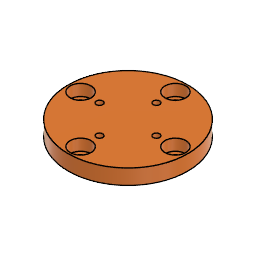
Assembly (Autodesk Fusion 360 archive; units mm, degrees)
design "Franka / UR10 mount"
part number: 2026-03-03-19-08-19-558
Autodesk Fusion 360 part; units mm, degrees
sketch "Sketch1" plane through (0, 0, 0) normal (0, 0, 1) x (1, 0, 0)
  circle A0 centre (0, 0) radius 15 construction
  circle A1 centre (0, 15) radius 1.7
  circle A2 centre (-15, 0) radius 1.7
  circle A3 centre (0, -15) radius 1.7
  circle A4 centre (15, 0) radius 1.7
  circle A5 centre (0, 0) radius 25
  circle A6 centre (0, 25) radius 1.5 construction
  circle A7 centre (-25, 0) radius 1.5 construction
  circle A8 centre (0, -25) radius 1.5 construction
  circle A9 centre (25, 0) radius 1.5 construction
  circle A10 centre (0, 0) radius 31.5
  circle A11 centre (0, 0) radius 25 construction
  dimension "d426" = 30
  dimension "d427" = 3.4
  dimension "d429" = 360
  dimension "d430" = 50
  dimension "d432" = 3
  dimension "d442" = 63
  dimension "d443" = 50
  constraint coincident A0.centre A5.centre
  constraint coincident A0 A1.centre
  constraint concentric A0 A5
  constraint coincident A5 A6.centre
  constraint concentric A5 A10
  constraint concentric A5 A11
  measures "d426" diameter of A0
  measures "d427" diameter of A1
  measures "d430" diameter of A5
  measures "d432" diameter of A6
  measures "d442" diameter of A10
  measures "d443" diameter of A11
extrude "Extrude1" add sketch "Sketch1" along normal blind 8 contours A5 | A10
hole "Hole2" at (15, 0, 0) at (0, -15, 0) at (-15, 0, 0) at (0, 15, 0) direction (0, 0, 1) diameter 3.4 depth 9 tip angle 118 counterbore diameter 6.5 counterbore depth 3
sketch "Sketch2" plane through (0, 0, 8) normal (0, 0, 1) x (-1, 0, 0)
  circle A0 centre (-15, 0) radius 1.7
  circle A1 centre (15, 0) radius 1.7
  circle A2 centre (0, 15) radius 1.7
  circle A3 centre (0, -15) radius 1.7
  circle A4 centre (0, 0) radius 31.5
  circle A5 centre (0, 0) radius 25
  circle A6 centre (0, -25) radius 1.5 construction
  circle A7 centre (25, 0) radius 1.5 construction
  circle A8 centre (0, 25) radius 1.5 construction
  circle A9 centre (-25, 0) radius 1.5 construction
  dimension "d449" = 50
  dimension "d450" = 3
  dimension "d452" = 360
  constraint coincident A4.centre A5.centre
  constraint coincident A5 A6.centre
  measures "d449" diameter of A5
  measures "d450" diameter of A6
hole "Hole3" at (0, 25, 8) at (25, 0, 8) at (0, -25, 8) at (-25, 0, 8) direction (0, 0, -1) diameter 6.6 depth 9 tip angle 118 counterbore diameter 11 counterbore depth 6
equation "d426 = promjer_utori"
equation "d443 = promjer_silikona"
equation "promjer_prihvata = promjer_silikona - 10 mm"
equation "promjer_silikona = 50 mm"
equation "promjer_utori = promjer_prihvata - 10 mm"
named bodies: "Franka prihvat"

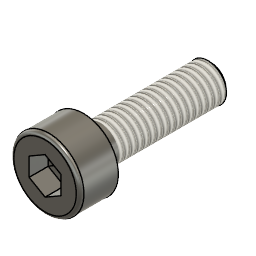
design "Broached Hexagon Socket Head Cap Screw ASME B18.3.1M - M3x0.5 x 10 Steel Grade 2 Plain"
description: Broached Hexagon Socket Head Cap Screw ASME B18.3.1M - M3x0.5 x 10
part number: BSHCS ASME B18.3.1M - M3x0.5 x 10 Steel Grade 2 Plain
Autodesk Fusion 360 part; units mm, degrees
sketch "Sketch1" plane through (0, 0, 0) normal (0, 1, 0) x (1, 0, 0)
  line L0 (-1.5, 0) -> (-1.5, 10)
  line L1 (-1.5, 10) -> (0, 10)
  line L2 (0, 10) -> (0, -3)
  line L3 (-1.5, 0) -> (-2.75, 0)
  line L4 (-2.75, 0) -> (-2.75, -3)
  line L5 (-2.75, -3) -> (0, -3)
  dimension "d101" = 10
  dimension "d102" = 3
  dimension "d109" = 5.5
  dimension "d110" = 3
  constraint perpendicular L0 L1
  constraint collinear origin L1.end L2.end
  constraint perpendicular L0 L3
  constraint coincident origin L3
  constraint vertical L2
  constraint coincident L2 L5.end
  constraint perpendicular L2 L5
  measures "d101" distance of origin L1
  measures "d102" distance of L3.end L5
revolve "Revolve1" add sketch "Sketch1" angle 360 about axis through (0, 0, -10) along (0, 0, 1)
ref_plane "WorkPlane1" through (0, 0, 3) normal (0, 0, 1) x (1, 0, 0)
sketch "Sketch6" plane through (0, 0, 3) normal (0, 0, 1) x (1, 0, 0)
  line L0 (0, -1.4434) -> (1.25, -0.7217)
  line L1 (1.25, -0.7217) -> (1.25, 0.7217)
  line L2 (1.25, 0.7217) -> (0, 1.4434)
  line L3 (0, 1.4434) -> (-1.25, 0.7217)
  line L4 (-1.25, 0.7217) -> (-1.25, -0.7217)
  line L5 (-1.25, -0.7217) -> (0, -1.4434)
  dimension "d111" = 2.5
  constraint vertical L1
  measures "d111" distance of L1 L4
extrude "Extrude1" cut sketch "Sketch6" against normal blind 1.5
extrude "Extrude2" cut 1 faces at (0.4167, -0.2406, 1.5) along direction (0, 0, -1) blind 1.5 draft -85
thread "Thread3" "ANSI Metric M Profile 3.0 M3x0.5 M3x0.5 4g6g" major diameter 2.927 minor diameter 2.369 pitch 0.5 angle 60 resizes the face on face at (-1.4925, 0.1494, -6.6667) from (0, 0, -1.3067) to (0, 0, -10)
fillet "Fillet4" radius 0.3 1 edges at (-2.5639, 0.9944, 3)
sketch "Sketch7" plane through (0, 0, 0) normal (0, 1, 0) x (1, 0, 0)
  line L0 (-1.53, 10) -> (-1.53, 9.6933)
  line L1 (-1.53, 9.6933) -> (-1.1933, 10)
  line L2 (0, 10) -> (0, -3)
  line L3 (-1.53, 10) -> (0, 10)
  dimension "d104" = 1.1933
  dimension "d105" = 1.53
  dimension "d106" = 0.3067
  constraint coincident L2.start L3.end
  constraint perpendicular L2 L3
  constraint coincident L1.end L3
  constraint perpendicular L0 L3
  measures "d104" distance of L1.end L2
  measures "d105" distance of L0 L2.start
  measures "d106" distance of L0.end L3
revolve "Revolve3" cut sketch "Sketch7" angle 360 about axis through (0, 0, 1.75) along (0, 0, 1)
equation "adsk_nomlen = 10.00 mm"
equation "adsk_headh = 3.00 mm"
equation "adsk_headdia = 5.50 mm"
equation "adsk_nomdia = 3.00 mm"
equation "adsk_philwidth = 2.50 mm"
equation "d31 = -adsk_phildepth"
equation "adsk_phildepth = 1.50 mm"
equation "d71 = adsk_headh"
equation "d76 = -adsk_phildepth"
equation "adsk_thrlen = 8.693275 mm"
equation "d86 = adsk_nomdia * 0.1"
equation "adsk_startlen = 0.306725 mm"
equation "adsk_endpointdia = 2.38655 mm"
equation "d101 = adsk_nomlen"
equation "d102 = adsk_headh"
equation "d104 = adsk_endpointdia / 2"
equation "d105 = adsk_nomdia * 0.51"
equation "d106 = adsk_startlen"
equation "d108 = min(adsk_thrlen; adsk_nomlen - 0.001 mm)"
equation "d109 = adsk_headdia"
equation "d110 = adsk_nomdia"
equation "d111 = adsk_philwidth"
